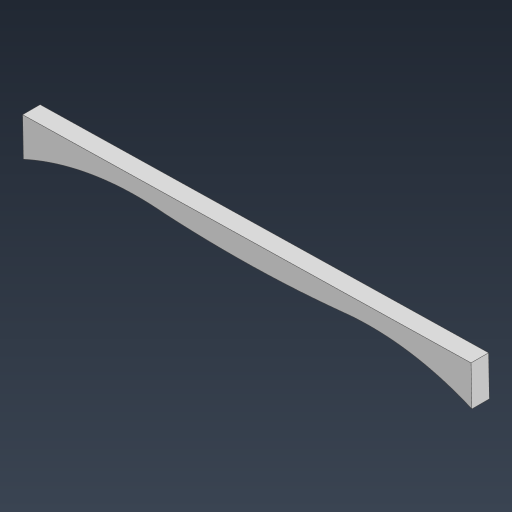
# Autodesk Inventor part: deseczka_dol_check
Saved by Autodesk Inventor 2023 (Build 270158000, 158)
## iProperties
Created: 2025-12-25
Part Number: deseczka_dol_check
Material: Generic
Document SubType Name: Modeling
Designer: szymo
Density: 1 g/cm^3
Appearance: Default
Author: szymo
Autodesk Inventor part; units mm, degrees
ref_plane "YZ Plane" through (0, 0, 0) normal (1, 0, 0) x (0, 1, 0)
ref_plane "XZ Plane" through (0, 0, 0) normal (0, 1, 0) x (-1, 0, 0)
ref_plane "XY Plane" through (0, 0, 0) normal (0, 0, 1) x (1, 0, 0)
sketch "Sketch1" plane through (0, 0, 0) normal (0, 0, 1) x (1, 0, 0)
  line L0 (0, 0) -> (293.4944, 0) construction
  line L1 (293.4944, 0) -> (293.4944, -132.0217) construction
  line L2 (293.4944, -132.0217) -> (0, -132.0217) construction
  line L3 (0, -132.0217) -> (0, 0) construction
  line L4 (79.3681, -56.3049) -> (159.3681, -56.3049) construction
  line L5 (283.1562, -93.1287) -> (278.6861, -90.8884) construction
  line L6 (283.1562, -93.1287) -> (282.3201, -93.1287) construction
  line L7 (18.3483, -97.5091) -> (22.8892, -95.4163) construction
  line L8 (18.3483, -97.5091) -> (20.5956, -97.5091) construction
  arc A0 (103.0994, -81.9859) -> (22.8892, -95.4163) centre (88.0559, -238.3753) ccw
  arc A1 (278.6861, -90.8884) -> (204.4098, -79.893) centre (221.0301, -223.9922) ccw
  arc A2 (103.0994, -81.9859) -> (204.4098, -79.893) centre (140.8276, 544.7964) ccw
  line L9 (22.8892, -95.4163) -> (22.4395, -73.648)
  line L10 (22.4395, -73.648) -> (278.2208, -68.3638)
  line L11 (278.2208, -68.3638) -> (278.6861, -90.8884)
  line L12 (103.0994, -81.9859) -> (204.4098, -79.893)
  line L13 (103.0994, -81.9859) -> (102.8928, -71.9859)
  line L14 (204.4098, -79.893) -> (204.2032, -69.893)
  dimension "d5" = 80
  dimension "d85" = 5
  dimension "d87" = 26.619
  dimension "d92" = 5
  dimension "d94" = 24.743
  dimension "d100" = 30
  dimension "d101" = 30
  dimension "d119" = 10
  dimension "d122" = 9.256
  constraints: 22 end point, 6 point on circle, 5 horizontal, 3 centre point, 3 parallel, 2 perpendicular, 2 point on line, 7 other
  measures "d5" distance of L4.start L4.end
  measures "d85" distance of L5.start L5.end
  measures "d87" angle of L5 L6
  measures "d92" distance of L7.start L7.end
  measures "d94" angle of L7 L8
  measures "d119" vertical distance of L12.start L13.end
extrude "Extrusion1" add sketch "Sketch1" along normal blind 10
body "Solid1"
